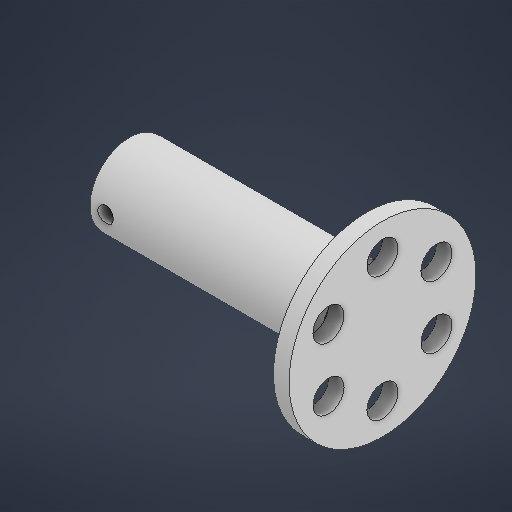
# Autodesk Inventor part: Hub-CV Adapter
Saved by Autodesk Inventor 2026.1 (Build 301233000, 233)
## iProperties
Created: 2026-06-12
Part Number: Hub-CV Adapter
Material: Generic
Document SubType Name: Modeling
Designer: share
Density: 1 g/cm^3
Appearance: Default
Author: share
Autodesk Inventor part; units mm, degrees
ref_plane "YZ Plane" through (0, 0, 0) normal (1, 0, 0) x (0, 1, 0)
ref_plane "XZ Plane" through (0, 0, 0) normal (0, 1, 0) x (-1, 0, 0)
sketch "Sketch1" plane through (0, 0, 0) normal (1, 0, 0) x (0, 1, 0)
  circle A0 centre (0, 0) radius 8.89
  circle A1 centre (0, 0) radius 12.7
  dimension "d0" = 25.4
  dimension "d1" = 3.81
  constraints: 2 centre point, 2 coincident
  measures "d0" diameter of A1
  measures "d1" radial gap between concentric circles of A1 A0
extrude "Main Shaft" add sketch "Sketch1" against normal blind 76.2
sketch "Sketch2" plane through (0, 0, 0) normal (1, 0, 0) x (0, 0, -1)
  circle A0 centre (0, 0) radius 30
  dimension "d4" = 60
  constraints: 1 centre point, 1 coincident
  measures "d4" diameter of A0
extrude "CV Flange" add sketch "Sketch2" along normal blind 5
sketch "Sketch3" plane through (5, 0, 0) normal (1, 0, 0) x (0, 0, -1)
  circle A0 centre (0, 20) radius 5
  circle A1 centre (0, 0) radius 20 construction
  line L0 (0, 0) -> (0, 20) construction
  dimension "d7" = 40
  dimension "d8" = 10
  constraints: 2 end point, 1 centre point, 1 coincident, 1 vertical, 1 vertical alignment, 2 other
  measures "d8" diameter of A0
extrude "CV Bolt Hole" cut sketch "Sketch3" against normal up to surface (5 mm away)
pattern_circular "CV Bolt Pattern" count 6 over 360 about axis through (-10, 0, 0) along (1, 0, 0) of "CV Bolt Hole"
chamfer "Weld_Chamfer" distance 2 angle 45 1 edges at (0, -12.7, 0)
ref_plane "Lock Pin Hole Plane" through (0, 0, 12.7) normal (0, 0, 1) x (1, 0, 0)
sketch "Sketch4" plane through (0, 0, 12.7) normal (0, 0, 1) x (1, 0, 0)
  line L0 (-76.2, 12.7) -> (-76.2, -12.7) projected
  line L1 (-2, -12.7) -> (-2, 12.7) projected
  circle A0 centre (-71.2, 0) radius 2.5
  point P0 (0, 0)
  dimension "d19" = 5
  dimension "d20" = 5
  constraints: 1 centre point
  measures "d19" distance from line of L0 A0.centre
  measures "d20" diameter of A0
extrude "Lock Pin Hole" cut sketch "Sketch4" against normal through all
equation "\"d0\" = Shaft_Diameter"
equation "\"d1\" = Shaft_Wall_Thickness"
equation "\"d4\" = Driveshaft_Flange_Diameter"
equation "\"d5\" = Driveshaft_Flange_Thickness"
equation "\"d7\" = CV_Bolt_Pattern_Diameter"
equation "\"d8\" = CV_Bolt_Hole_Diameter"
equation "\"d19\" = Hub_Lock_Pin_Edge_Distance"
equation "\"d20\" = Hub_Lock_Pin_Hole_Diameter"
equation "\"Shaft_Diameter\" = 25.4"
equation "\"Shaft_Wall_Thickness\" = 3.81"
equation "\"Driveshaft_Flange_Diameter\" = 60"
equation "\"Driveshaft_Flange_Thickness\" = 5"
equation "\"CV_Bolt_Hole_Diameter\" = 10"
equation "\"d18\" = 0.5 * Shaft_Diameter"
equation "\"Hub_Lock_Pin_Hole_Diameter\" = 5"
equation "\"Hub_Lock_Pin_Edge_Distance\" = 5"
equation "\"CV_Bolt_Pattern_Diameter\" = 40"
body "Solid1"
